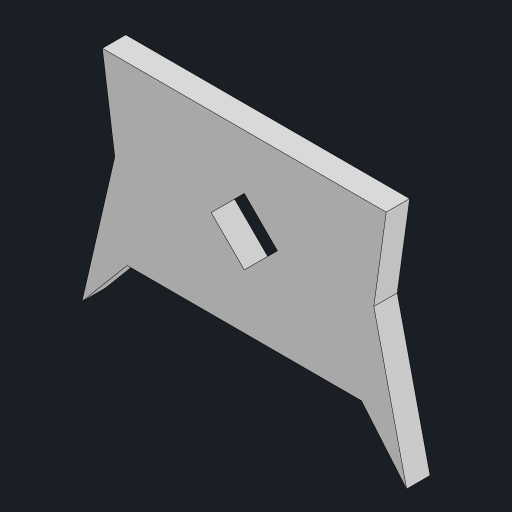
# Autodesk Inventor part: om_BackHolder_V2
Saved by Autodesk Inventor 2023 (Build 270158000, 158)
## iProperties
Created: 2022-07-14
Part Number: om_BackHolder_V2
Material: 一般
Document SubType Name: Modeling
Designer: legot
Density: 1 g/cm^3
Appearance: 既定
Author: legot
Autodesk Inventor part; units mm, degrees
ref_plane "YZ Plane" through (0, 0, 0) normal (1, 0, 0) x (0, 1, 0)
ref_plane "XZ Plane" through (0, 0, 0) normal (0, 1, 0) x (-1, 0, 0)
ref_plane "XY Plane" through (0, 0, 0) normal (0, 0, 1) x (1, 0, 0)
sketch "スケッチ1" plane through (0, 0, 0) normal (0, 0, 1) x (1, 0, 0)
  line L0 (2.8284, 0) -> (0, -2.8284)
  line L1 (0, -2.8284) -> (-2.8284, 0)
  line L2 (-2.8284, 0) -> (0, 2.8284)
  line L3 (0, 2.8284) -> (2.8284, 0)
  line L4 (-12.1149, 7.5) -> (-10, -7.5)
  line L5 (10, -7.5) -> (-10, -7.5)
  line L6 (10, -7.5) -> (12.1149, 7.5)
  line L7 (12.1149, 7.5) -> (-12.1149, 7.5)
  point P0 (0, 0)
  point P1 (0, 7.5)
  point P2 (11.0574, 0)
  dimension "d10" = 24.2298
  dimension "d11" = 20
  dimension "d12" = 15
  dimension "d13" = 4
  constraints: 16 end point, 4 equal length, 3 vertical alignment, 2 horizontal alignment, 2 midpoint, 1 horizontal, 1 perpendicular
  measures "d10" distance of L6.end L4.start
  measures "d11" distance of L5.start L4.end
  measures "d12" distance between parallel lines of L7 L5
  measures "d13" distance of L2.end L0.start
extrude "押し出し1" add sketch "スケッチ1" against normal blind 2
sketch "スケッチ2" plane through (0, 0, 0) normal (0, 0, 1) x (1, 0, 0)
  line L0 (10, -7.5) -> (13.8567, -12.0963)
  line L1 (13.8567, -12.0963) -> (11.0574, 0)
  line L2 (-12.1149, 7.5) -> (12.1149, 7.5) projected
  line L3 (12.1149, 7.5) -> (10, -7.5) projected
  line L4 (10, -7.5) -> (-10, -7.5) projected
  line L5 (-10, -7.5) -> (-12.1149, 7.5) projected
  line L6 (0, -2.8284) -> (2.8284, 0) projected
  line L7 (2.8284, 0) -> (0, 2.8284) projected
  line L8 (0, 2.8284) -> (-2.8284, 0) projected
  line L9 (-2.8284, 0) -> (0, -2.8284) projected
  dimension "d7" = 6
  dimension "d14" = 130
  constraints: 4 end point, 2 midpoint
  measures "d7" distance of L0.start L0.end
  measures "d14" angle of L0 L4
extrude "押し出し2" add sketch "スケッチ2" against normal up to surface (2 mm away) contours L3 L1 L0
mirror "ミラー1" about plane through (0, 0, 0) normal (1, 0, 0) of "押し出し2"
